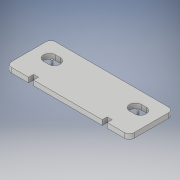
# Autodesk Inventor part: Gantry side load
Saved by Autodesk Inventor 2018.2 (Build 222227000, 227)
## iProperties
Created: 2017-12-19
Part Number: Gantry side load
Material: Generic
Document SubType Name: Modeling
Designer: torba
Density: 1 g/cm^3
Appearance: Default
Author: torba
Autodesk Inventor part; units mm, degrees
ref_plane "YZ Plane" through (0, 0, 0) normal (1, 0, 0) x (0, 1, 0)
ref_plane "XZ Plane" through (0, 0, 0) normal (0, 1, 0) x (-1, 0, 0)
ref_plane "XY Plane" through (0, 0, 0) normal (0, 0, 1) x (1, 0, 0)
sketch "Sketch1" plane through (0, 0, 0) normal (0, 1, 0) x (-1, 0, 0)
  line L0 (0, 0) -> (28.575, 0)
  line L1 (28.575, 0) -> (34.925, 0)
  line L2 (34.925, 0) -> (123.825, 0)
  line L3 (123.825, 0) -> (130.175, 0)
  line L4 (130.175, 0) -> (158.75, 0)
  line L5 (158.75, 0) -> (158.75, -12.7)
  line L6 (158.75, -12.7) -> (0, -12.7)
  line L7 (0, -12.7) -> (0, 0)
  line L8 (28.575, 0) -> (28.575, -12.7)
  line L9 (34.925, 0) -> (34.925, -12.7)
  line L10 (123.825, 0) -> (123.825, -12.7)
  line L11 (130.175, 0) -> (130.175, -12.7)
  line L12 (0, -12.7) -> (0, -57.15)
  line L13 (0, -57.15) -> (158.75, -57.15)
  line L14 (158.75, -57.15) -> (158.75, -12.7)
  dimension "d73" = 28.575
  dimension "d74" = 6.35
  dimension "d75" = 88.9
  dimension "d76" = 6.35
  dimension "d77" = 28.575
  dimension "d78" = 12.7
  dimension "d79" = 44.45
  constraints: 30 end point, 10 point on line, 7 perpendicular, 1 horizontal, 1 parallel
  measures "d73" distance of L0.start L0.end
  measures "d74" distance of L0.end L1.end
  measures "d75" distance of L1.end L2.end
  measures "d76" distance of L2.end L3.end
  measures "d77" distance of L3.end L4.end
  measures "d78" distance of L4.end L5.end
  measures "d79" distance of L6.end L12.end
extrude "Extrusion10" add sketch "Sketch1" against normal blind 6.35 contours L0 L8 L6 L7 | L6 L14 L13 L12 | L2 L10 L6 L9 | L4 L5 L6 L11
sketch "Sketch7" plane through (0, -6.35, 0) normal (0, -1, 0) x (1, 0, 0)
  line L0 (-130.175, -12.7) -> (-130.175, 0) projected
  line L1 (-130.175, 0) -> (-158.75, 0) projected
  line L2 (-158.75, 0) -> (-158.75, -57.15) projected
  line L3 (-158.75, -57.15) -> (0, -57.15) projected
  line L4 (0, -57.15) -> (0, 0) projected
  line L5 (0, 0) -> (-28.575, 0) projected
  line L6 (-28.575, 0) -> (-28.575, -12.7) projected
  line L7 (-28.575, -12.7) -> (-34.925, -12.7) projected
  line L8 (-34.925, -12.7) -> (-34.925, 0) projected
  line L9 (-34.925, 0) -> (-123.825, 0) projected
  line L10 (-123.825, 0) -> (-123.825, -12.7) projected
  line L11 (-123.825, -12.7) -> (-130.175, -12.7) projected
  line L12 (-28.575, -12.7) -> (-34.925, -12.7) projected
  line L13 (-158.75, -57.15) -> (0, -57.15) projected
  line L14 (0, -57.15) -> (0, 0) projected
  line L15 (0, -34.925) -> (-158.75, -34.925) construction
  line L16 (-158.75, 0) -> (-158.75, -57.15) projected
  line L17 (-34.925, -12.7) -> (-34.925, 0) projected
  line L18 (-34.925, -12.7) -> (-41.275, -12.7) construction
  line L19 (-123.825, -12.7) -> (-117.475, -12.7) construction
  line L20 (-117.475, -12.7) -> (-117.475, -34.925) construction
  line L21 (-41.275, -12.7) -> (-41.275, -34.925) construction
  line L22 (-41.275, -34.925) -> (-26.95, -34.925) construction
  line L23 (-117.475, -34.925) -> (-131.8, -34.925) construction
  line L24 (-26.95, -34.925) -> (-20.6, -34.925)
  line L25 (-131.8, -34.925) -> (-138.15, -34.925)
  line L26 (-131.8, -34.925) -> (-138.15, -34.925) construction
  line L27 (-131.8, -27.425) -> (-138.15, -27.425)
  line L28 (-138.15, -42.425) -> (-131.8, -42.425)
  arc A0 (-131.8, -42.425) -> (-131.8, -27.425) centre (-131.8, -34.925) ccw
  arc A1 (-138.15, -27.425) -> (-138.15, -42.425) centre (-138.15, -34.925) ccw
  line L29 (-20.6, -34.925) -> (-26.95, -34.925) construction
  line L30 (-20.6, -27.425) -> (-26.95, -27.425)
  line L31 (-26.95, -42.425) -> (-20.6, -42.425)
  arc A2 (-20.6, -42.425) -> (-20.6, -27.425) centre (-20.6, -34.925) ccw
  arc A3 (-26.95, -27.425) -> (-26.95, -42.425) centre (-26.95, -34.925) ccw
  circle A4 centre (-20.6, -34.925) radius 17.5 construction
  circle A5 centre (-138.15, -34.925) radius 17.5 construction
  point P0 (-134.975, -34.925)
  point P1 (-23.775, -34.925)
  dimension "d83" = 6.35
  dimension "d84" = 6.35
  dimension "d85" = 22.225
  dimension "d86" = 14.325
  dimension "d87" = 14.325
  dimension "d88" = 6.35
  dimension "d89" = 6.35
  dimension "d90" = 15
  dimension "d91" = 15
  dimension "d92" = 35
  dimension "d93" = 35
  constraints: 34 end point, 8 point on circle, 8 point on line, 8 tangent, 6 centre point, 2 coincident, 2 collinear, 2 horizontal, 2 midpoint, 2 parallel, 2 perpendicular
  measures "d83" distance of L7.end L18.end
  measures "d84" distance of L10.end L19.end
  measures "d85" distance between parallel lines of L3 L15
  measures "d86" distance of L21.end L22.end
  measures "d87" distance of L20.end L23.end
  measures "d88" distance of L22.end L24.end
  measures "d89" distance of L23.end L25.end
  measures "d90" diameter of A1
  measures "d91" diameter of A3
  measures "d92" diameter of A4
  measures "d93" diameter of A5
extrude "Extrusion11" cut sketch "Sketch7" against normal blind 6.35 contours A0 L28 A1 L27 | A2 L31 A3 L30
fillet "Fillet4" radius 6.35 4 edges at (0, -3.175, 0) (0, -3.175, -57.15) (-158.75, -3.175, -57.15) (-158.75, -3.175, 0)
sketch "Sketch9" plane through (0, 0, 0) normal (0, 1, 0) x (1, 0, 0)
  line L0 (-138.15, 42.425) -> (-131.8, 42.425) projected
  line L1 (-131.8, 27.425) -> (-138.15, 27.425) projected
  line L2 (-26.95, 42.425) -> (-20.6, 42.425) projected
  line L3 (-20.6, 27.425) -> (-26.95, 27.425) projected
  line L4 (-131.8, 42.425) -> (-138.15, 42.425) projected
  line L5 (-134.975, 42.425) -> (-134.975, 27.425)
  line L6 (-20.6, 42.425) -> (-26.95, 42.425) projected
  line L7 (-23.775, 42.425) -> (-23.775, 27.425)
  circle A0 centre (-134.975, 34.925) radius 1.27
  circle A1 centre (-23.775, 34.925) radius 1.27
  point P0 (0, 0)
  dimension "d97" = 2.54
  dimension "d98" = 2.54
  constraints: 6 midpoint, 4 end point, 2 centre point
  measures "d97" diameter of A0
  measures "d98" diameter of A1
extrude "Extrusion12" add sketch "Sketch9" against normal up to surface (6.35 mm away) separate body
sketch "Sketch10" plane through (-130.175, 0, -12.7) normal (0, 0, 1) x (1, 0, 0)
  line L0 (0, 0) -> (6.35, 0) projected
  line L1 (6.35, -6.35) -> (0, -6.35) projected
  line L2 (6.35, 0) -> (6.35, -6.35) projected
  line L3 (0, 0) -> (0, -6.35) projected
  line L4 (95.25, 0) -> (101.6, 0) projected
  line L5 (101.6, 0) -> (101.6, -6.35) projected
  line L6 (101.6, -6.35) -> (95.25, -6.35) projected
  line L7 (95.25, 0) -> (95.25, -6.35) projected
  point P0 (130.175, 0)
extrude "Extrusion13" add sketch "Sketch10" along normal blind 6.35 bodies 1
body "Solid2"
body "Solid3"
